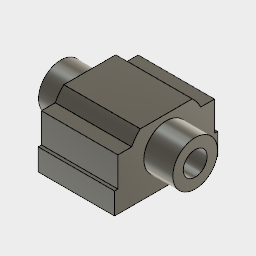
Base_v7 (Autodesk Fusion 360 archive; units mm, degrees)
design "Y Axis Bearing Block"
Autodesk Fusion 360 part; units mm, degrees
note: some values were not read from the file. Chosen so that the rebuilt part matches the saved one: how an offset face is resized.
sketch "Base" plane through (0, 0, 0) normal (0, 0, 1) x (1, 0, 0) in component "X Bearing Blocks"
  line L0 (12.8, 17.3) -> (-12.8, 17.3)
  line L1 (-12.8, 17.3) -> (-12.8, -17.3)
  line L2 (-12.8, -17.3) -> (12.8, -17.3)
  line L3 (12.8, -17.3) -> (12.8, 17.3)
  line L4 (12.8, 17.3) -> (-12.8, -17.3) construction
  line L5 (-12.8, 17.3) -> (12.8, -17.3) construction
  line L6 (-12.8, 0) -> (12.8, 0) construction
  line L7 (-12.8, 14.125) -> (12.8, 14.125)
  line L8 (-12.8, 9.875) -> (12.8, 9.875)
  line L9 (-12.8, 12) -> (12.8, 12) construction
  circle A0 centre (-8.5, 12) radius 2
  circle A1 centre (8.5, 12) radius 2
  line L10 (0, 17.3) -> (0, -17.3) construction
  line L11 (-12.8, -14.125) -> (12.8, -14.125)
  circle A2 centre (-8.5, -12) radius 2
  circle A3 centre (8.5, -12) radius 2
  line L12 (-12.8, -9.875) -> (12.8, -9.875)
  dimension "d484_1" = 25.6
  dimension "d485_1" = 34.6
  dimension "d489_1" = 4
  dimension "d490_1" = 4
  dimension "d491_1" = 12
  dimension "d492_1" = 17
  dimension "d493_1" = 8.5
  dimension "d495_1" = 2.125
  dimension "d496_1" = 2.125
  measures "d484_1" distance of L1.end L2.end
  measures "d485_1" distance of L0.end L1.end
  measures "d489_1" diameter of A0
  measures "d490_1" diameter of A1
  measures "d491_1" distance of L6 L9
  measures "d492_1" distance of A0.centre A1.centre
  measures "d493_1" distance of A0.centre L10
  measures "d495_1" distance of L8 L9
  measures "d496_1" distance of L7 L9
extrude "Extrude1" add sketch "Base" along normal blind 21 contours L0 L1 L3 L7 | L1 L3 L7 L8 | L1 L3 L8 L12 | L1 L3 L11 L12 | L1 L2 L3 L11 | A0 | A1 | A2 | A3 in component "X Bearing Blocks"
sketch "Face" plane through (12.8, 0, 0) normal (1, 0, 0) x (0, 1, 0) in component "X Bearing Blocks"
  line L0 (-17.3, 0) -> (17.3, 0)
  line L1 (17.3, 0) -> (17.3, 21)
  line L2 (17.3, 21) -> (-17.3, 21)
  line L3 (-17.3, 21) -> (-17.3, 0)
  line L4 (0, 0) -> (0, 21) construction
  circle A0 centre (0, 11.5) radius 7.5
  circle A1 centre (0, 11.5) radius 4
  line L5 (-17.3, 0) -> (-17.3, 7.3)
  line L6 (-17.3, 7.3) -> (-16.2, 7.3)
  line L7 (-16.2, 7.3) -> (-16.2, 17.2)
  line L8 (-16.2, 17.2) -> (-11.55, 17.2)
  line L9 (17.3, 0) -> (17.3, 7.3)
  line L10 (17.3, 7.3) -> (16.2, 7.3)
  line L11 (16.2, 7.3) -> (16.2, 17.2)
  line L12 (16.2, 17.2) -> (11.55, 17.2)
  arc A2 (11.55, 17.2) -> (-11.55, 17.2) centre (0, 11.5) ccw
  dimension "d499_1" = 15
  dimension "d500_1" = 8
  dimension "d501_1" = 11.5
  dimension "d504_1" = 1.1
  dimension "d505_1" = 7.3
  dimension "d506_1" = 5.75
  dimension "d507_1" = 17.2
  measures "d499_1" diameter of A0
  measures "d500_1" diameter of A1
  measures "d501_1" distance of L0 A0.centre
  measures "d504_1" distance of L5.end L6.end
  measures "d505_1" distance of L0.start L5.end
  measures "d506_1" distance of L3 L8.end
  measures "d507_1" distance of L0 L8
extrude "Extrude2" cut sketch "Face" against normal blind 25.6 contours L2 L3 L6 L7 L8 A2 | L1 L2 L10 L11 L12 A2 | A1 in component "X Bearing Blocks"
extrude "Extrude3" add sketch "Face" along normal mid plane 45 from surface at -12.8 contours A0 in component "X Bearing Blocks"
extrude "Extrude4" cut sketch "Base" along normal blind 4 contours A0 | A1 | A2 | A3 in component "X Bearing Blocks"
thread "Thread1" "ISO Metric profile 4.0 M4x0.7 6H" major diameter 4.1095 minor diameter 3.332 pitch 0.7 angle 60 resizes the face on face at (-6.5025, -12.0997, 2.6667) in component "X Bearing Blocks"
thread "Thread2" "ISO Metric profile 4.0 M4x0.7 6H" major diameter 4.1095 minor diameter 3.332 pitch 0.7 angle 60 resizes the face on face at (10.4901, -11.8009, 2.6667) in component "X Bearing Blocks"
thread "Thread3" "ISO Metric profile 4.0 M4x0.7 6H" major diameter 4.1095 minor diameter 3.332 pitch 0.7 angle 60 resizes the face on face at (10.4901, 12.1991, 2.6667) in component "X Bearing Blocks"
thread "Thread4" "ISO Metric profile 4.0 M4x0.7 6H" major diameter 4.1095 minor diameter 3.332 pitch 0.7 angle 60 resizes the face on face at (-6.5099, 12.1991, 2.6667) in component "X Bearing Blocks"
component "X Bearing Blocks" placed x (1, 0, 0) y (0, 1, 0) z (0, 0, 1) at (0, 0, 0)
equation "d197_1 = 4 mm"
equation "d198_1 = 6.00 mm"
equation "d199_1 = 6.00 mm"
equation "d200_1 = 4.00 mm"
equation "d201_1 = 12 mm"
equation "d202_1 = 90.0 deg"
equation "d203_1 = 12 mm"
equation "d204_1 = 90.0 deg"
equation "d205_1 = 12 mm"
equation "d206_1 = 90.0 deg"
equation "d207_1 = 51 mm"
equation "d209_1 = 51 mm"
equation "d210_1 = 12 mm"
equation "d211_1 = 90.0 deg"
equation "d212_1 = 30.0 mm"
equation "d213_1 = 30.00 mm"
equation "d214_1 = 12 mm"
equation "d215_1 = 90.0 deg"
equation "d216_1 = 12 mm"
equation "d217_1 = 90.0 deg"
equation "d218_1 = 2 mm"
equation "d225_1 = ( 3.6 / 2 ) * 1 mm"
equation "d227_1 = -1.5875 mm"
equation "d228_1 = 0.0 deg"
equation "d229_1 = 5.00 mm"
equation "d250_1 = 1.5875 mm"
equation "d251_1 = 0.0 deg"
equation "d253_1 = 21 mm + ( ( 39 / 2 ) * 1 mm )"
equation "d260_1 = 360.0 deg"
equation "d261_1 = -1.5875 mm"
equation "d262_1 = 0.0 deg"
equation "d284_1 = -1.588 mm"
equation "d285_1 = 0.0 deg"
equation "d286_1 = 0.00 mm"
equation "d287_1 = 1.588 mm"
equation "d288_1 = 0.0 deg"
equation "d301_1 = -1.588 mm"
equation "d302_1 = 0.0 deg"
equation "d342_1 = ( 17 / 2 ) * 1 mm"
equation "d343_1 = ( 17 / 2 ) * 1 mm"
equation "d386_1 = 0.00 mm"
equation "d387_1 = 19.7 mm"
equation "d388_1 = 0.0 deg"
equation "d389_1 = 0.00 mm"
equation "d390_1 = 6 mm"
equation "d391_1 = 0.0 deg"
equation "d400_1 = ( 92 / 2 ) * 1 mm"
equation "d407_1 = 0.00 mm"
equation "d408_1 = 9 mm"
equation "d409_1 = 0.0 deg"
equation "d410_1 = 1.588 mm"
equation "d411_1 = 0.0 deg"
equation "d433_1 = ( 92 / 2 ) * 1 mm"
equation "d448_1 = 0.00 mm"
equation "d449_1 = 0.00 mm"
equation "d450_1 = 0.00 mm"
equation "d451_1 = 0.0 deg"
equation "d452_1 = 0.00 mm"
equation "d453_1 = 0.00 mm"
equation "d454_1 = 0.00 mm"
equation "d455_1 = 0.0 deg"
equation "d456_1 = 90 deg"
equation "d457_1 = 0.00 mm"
equation "d458_1 = 0.00 mm"
equation "d459_1 = 0.00 mm"
equation "d460_1 = 0.00 mm"
equation "d461_1 = 0.00 mm"
equation "d462_1 = 0.00 mm"
equation "d463_1 = 0.0 deg"
equation "d464_1 = 0.00 mm"
equation "d465_1 = 0.00 mm"
equation "d466_1 = 0.00 mm"
equation "d467_1 = 0.0 deg"
equation "d468_1 = -90 deg"
equation "d469_1 = 0.00 mm"
equation "d470_1 = 0.00 mm"
equation "d471_1 = 0.00 mm"
equation "d491_1 = ( 24 / 2 ) * 1 mm"
equation "d493_1 = ( 17 / 2 ) * 1 mm"
equation "d495_1 = ( 4.25 / 2 ) * 1 mm"
equation "d496_1 = ( 4.25 / 2 ) * 1 mm"
equation "d497_1 = 21 mm"
equation "d498_1 = 0.0 deg"
equation "d501_1 = ( 15 / 2 ) * 1 mm + 4 mm"
equation "d508_1 = 0.0 deg"
equation "d509_1 = -25.60 mm"
equation "d510_1 = ( 45 / 2 ) * 1 mm"
equation "d511_1 = 0.0 deg"
equation "d512_1 = 0.00 mm"
equation "d513_1 = 4.00 mm"
equation "d514_1 = 0.0 deg"
equation "d515_1 = 0.00 mm"
equation "d516_1 = 0.00 mm"
equation "d517_1 = 0.00 mm"
equation "d518_1 = 0.0 deg"
equation "d519_1 = 0.00 mm"
equation "d520_1 = 0.00 mm"
equation "d521_1 = 0.00 mm"
equation "d522_1 = 0.0 deg"
equation "d523_1 = 90 deg"
equation "d524_1 = 0.00 mm"
equation "d525_1 = 0.00 mm"
equation "d526_1 = 0.00 mm"
equation "d527_1 = 0.00 mm"
equation "d528_1 = 0.00 mm"
equation "d529_1 = 0.00 mm"
equation "d530_1 = 0.0 deg"
equation "d531_1 = 0.00 mm"
equation "d532_1 = 0.00 mm"
equation "d533_1 = 0.00 mm"
equation "d534_1 = 0.0 deg"
equation "d535_1 = 90 deg"
equation "d536_1 = 0.00 mm"
equation "d537_1 = 0.00 mm"
equation "d538_1 = 0.00 mm"
equation "d539_1 = 0.00 mm"
equation "d540_1 = 0.00 mm"
equation "d541_1 = 0.00 mm"
equation "d542_1 = 0.0 deg"
equation "d543_1 = 0.00 mm"
equation "d544_1 = 0.00 mm"
equation "d545_1 = 0.00 mm"
equation "d546_1 = 0.0 deg"
equation "d547_1 = 0.0 deg"
equation "d548_1 = 0.00 mm"
equation "d549_1 = 0.00 mm"
equation "d550_1 = 0.00 mm"
equation "d587_1 = 0.00 mm"
equation "d588_1 = 0.00 mm"
equation "d589_1 = 0.00 mm"
equation "d590_1 = 0.0 deg"
equation "d491_1 = ( 24 / 2 ) * 1 mm"
equation "d493_1 = ( 17 / 2 ) * 1 mm"
equation "d495_1 = ( 4.25 / 2 ) * 1 mm"
equation "d496_1 = ( 4.25 / 2 ) * 1 mm"
equation "d501_1 = ( 15 / 2 ) * 1 mm + 4 mm"
equation "d510_1 = ( 45 / 2 ) * 1 mm"
